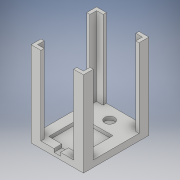
# Autodesk Inventor part: Part2
Saved by Autodesk Inventor 2019 (Build 230136000, 136)
## iProperties
Created: 2021-01-20
Part Number: Part2
Material: Generic
Document SubType Name: Modeling
Designer: kimsl
Density: 1 g/cm^3
Appearance: Default
Author: kimsl
Autodesk Inventor part; units mm, degrees
ref_plane "YZ Plane" through (0, 0, 0) normal (1, 0, 0) x (0, 1, 0)
ref_plane "XZ Plane" through (0, 0, 0) normal (0, 1, 0) x (-1, 0, 0)
ref_plane "XY Plane" through (0, 0, 0) normal (0, 0, 1) x (1, 0, 0)
sketch "Sketch1" plane through (0, 0, 0) normal (0, 1, 0) x (-1, 0, 0)
  line L0 (-40, 50) -> (40, 50)
  line L1 (40, 50) -> (40, -50)
  line L2 (40, -50) -> (-40, -50)
  line L3 (-40, -50) -> (-40, 50)
  line L4 (-40, 50) -> (40, -50) construction
  line L5 (40, 50) -> (-40, -50) construction
  point P0 (0, 0)
  dimension "d0" = 100
  dimension "d1" = 80
  constraints: 12 end point, 2 midpoint, 2 parallel, 1 horizontal, 1 perpendicular
  measures "d0" distance of L0.end L1.end
  measures "d1" distance of L1.end L2.end
extrude "Extrusion1" add sketch "Sketch1" along normal blind 10
sketch "Sketch2" plane through (0, 10, 0) normal (0, 1, 0) x (1, 0, 0)
  line L0 (-40, -50) -> (40, -50) projected
  line L1 (40, -50) -> (25, -50)
  line L2 (25, -50) -> (25, -35)
  line L3 (25, -35) -> (40, -35)
  line L4 (40, -35) -> (40, -50)
  line L5 (25, -35) -> (35, -35)
  line L6 (35, -35) -> (35, -45)
  line L7 (35, -45) -> (25, -45)
  line L8 (25, -45) -> (25, -35)
  point P0 (0, 0)
  dimension "d4" = 15
  dimension "d5" = 15
  dimension "d6" = 10
  dimension "d7" = 10
  constraints: 16 end point, 4 parallel, 2 horizontal, 2 perpendicular
  measures "d4" distance of L1.end L2.end
  measures "d5" distance of L2.end L3.end
  measures "d6" distance of L5.end L6.end
  measures "d7" distance of L6.end L7.end
extrude "Extrusion2" add sketch "Sketch2" along normal blind 120 contours L2 L7 L6 L3 L4 L0
mirror "Mirror1" about plane through (0, 0, 0) normal (0, 0, 1) of "Extrusion2"
mirror "Mirror2" about plane through (0, 0, 0) normal (1, 0, 0) of "Extrusion2", "Mirror1"
sketch "Sketch3" plane through (0, 10, 0) normal (0, 1, 0) x (1, 0, 0)
  line L0 (-25.02, -38.04) -> (23.02, -38.04)
  line L1 (23.02, -38.04) -> (23.02, 12)
  line L2 (23.02, 12) -> (-25.02, 12)
  line L3 (-25.02, 12) -> (-25.02, -38.04)
  line L4 (25, 50) -> (-25, 50) projected
  point P0 (0, 0)
  dimension "d10" = 48.04
  dimension "d11" = 50.04
  dimension "d13" = 25.02
  dimension "d14" = 38
  constraints: 8 end point, 2 parallel, 1 horizontal, 1 perpendicular
  measures "d10" distance of L0.start L0.end
  measures "d11" distance of L2.end L0.start
  measures "d13" distance from line of point (0, 0) L3
  measures "d14" distance between parallel lines of L4 L2
extrude "Extrusion3" cut sketch "Sketch3" against normal blind 5.04
sketch "Sketch4" plane through (0, 10, 0) normal (0, 1, 0) x (1, 0, 0)
  circle A0 centre (0, 30) radius 7.52
  line L0 (25, 50) -> (-25, 50) projected
  line L1 (-40, 35) -> (-40, -35) projected
  point P0 (0, 0)
  dimension "d17" = 15.04
  dimension "d18" = 20
  dimension "d19" = 40
  constraints: 1 centre point
  measures "d17" diameter of A0
  measures "d18" distance from line of L0 A0.centre
  measures "d19" distance from line of L1 A0.centre
extrude "Extrusion4" cut sketch "Sketch4" against normal blind 5.04
sketch "Sketch6" plane through (-40, 0, 50) normal (0, 0, 1) x (1, 0, 0)
  line L0 (63.02, 10) -> (14.98, 10) projected
  line L1 (65, 10) -> (65, 130) projected
  line L2 (35, 5) -> (45, 5)
  line L3 (45, 5) -> (45, 15)
  line L4 (45, 15) -> (35, 15)
  line L5 (35, 15) -> (35, 5)
  line L6 (35, 5) -> (45, 15) construction
  line L7 (45, 5) -> (35, 15) construction
  point P0 (40, 0)
  dimension "d24" = 10
  dimension "d25" = 10
  dimension "d26" = 20
  dimension "d27" = 5
  constraints: 12 end point, 2 parallel, 1 horizontal, 1 perpendicular
  measures "d24" distance of L3.end L4.end
  measures "d25" distance of L2.end L3.end
  measures "d26" distance between parallel lines of L1 L3
  measures "d27" distance between parallel lines of L0 L2
extrude "Extrusion5" cut sketch "Sketch6" against normal blind 15
body "Solid1"
